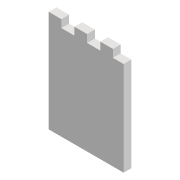
# Autodesk Inventor part: 00_Baseplate_Simmo_side6_v2
Saved by Autodesk Inventor 2022 (Build 260153000, 153)
## iProperties
Created: 2022-08-09
Part Number: 00_Baseplate_Simmo_side6_v2
Material: Generic
Document SubType Name: Modeling
Designer: wanghaoran
Density: 1 g/cm^3
Appearance: Default
Author: wanghaoran
Autodesk Inventor part; units mm, degrees
ref_plane "YZ Plane" through (0, 0, 0) normal (1, 0, 0) x (0, 1, 0)
ref_plane "XZ Plane" through (0, 0, 0) normal (0, 1, 0) x (-1, 0, 0)
ref_plane "XY Plane" through (0, 0, 0) normal (0, 0, 1) x (1, 0, 0)
sketch "Sketch1" plane through (0, 0, 0) normal (0, 0, 1) x (1, 0, 0)
  line L0 (40, 0) -> (48.2654, 0) projected
  line L1 (-10, 0) -> (-10, 6) projected
  line L2 (-10, 0) -> (-10, 6) projected
  line L3 (-10, 0) -> (-10, 6) projected
  line L4 (-10, 6) -> (48.2654, 6)
  line L5 (48.2654, 6) -> (48.2654, -73)
  line L6 (48.2654, -73) -> (-10, -73)
  line L7 (-10, -73) -> (-10, 6)
  point P0 (0, 0)
  dimension "d0" = 79
  constraints: 8 end point, 2 parallel, 1 horizontal, 1 perpendicular
  measures "d0" distance of L4.end L5.end
extrude "Extrusion1" add sketch "Sketch1" along normal blind 6
sketch "Sketch2" plane through (0, 0, 6) normal (0, 0, 1) x (1, 0, 0)
  line L0 (40, 0) -> (48.2654, 0) projected
  line L1 (40, 6) -> (40, 0) projected
  line L2 (48.2654, -73) -> (48.2654, 6) projected
  line L3 (48.2654, 6) -> (-10, 6) projected
  line L4 (20, 6) -> (20, 0) projected
  line L5 (10, 0) -> (10, 6) projected
  line L6 (0, 0) -> (10, 0) projected
  line L7 (0, 6) -> (0, 0) projected
  line L8 (20, 0) -> (30, 0) projected
  line L9 (30, 0) -> (30, 6) projected
  line L10 (40, 0) -> (39.9, 0)
  line L11 (39.9, 0) -> (39.9, 6)
  line L12 (39.9, 6) -> (40, 6)
  line L13 (40, 6) -> (40, 0)
  line L14 (30, 0) -> (30.1, 0)
  line L15 (30.1, 0) -> (30.1, 6)
  line L16 (30.1, 6) -> (30, 6)
  line L17 (30, 6) -> (30, 0)
  line L18 (20, 0) -> (19.9, 0)
  line L19 (19.9, 0) -> (19.9, 6)
  line L20 (19.9, 6) -> (20, 6)
  line L21 (20, 6) -> (20, 0)
  line L22 (10, 0) -> (10.1, 0)
  line L23 (10.1, 0) -> (10.1, 6)
  line L24 (10.1, 6) -> (10, 6)
  line L25 (10, 6) -> (10, 0)
  line L26 (0, 0) -> (-0.1, 0)
  line L27 (-0.1, 0) -> (-0.1, 6)
  line L28 (-0.1, 6) -> (0, 6)
  line L29 (0, 6) -> (0, 0)
  dimension "d3" = 0.1
  dimension "d4" = 6
  dimension "d5" = 0.1
  dimension "d6" = 6
  dimension "d7" = 0.1
  dimension "d8" = 6
  dimension "d9" = 0.1
  dimension "d10" = 6
  dimension "d11" = 0.1
  dimension "d12" = 6
  constraints: 40 end point, 10 parallel, 5 horizontal, 5 perpendicular
  measures "d3" distance of L11.end L12.end
  measures "d4" distance of L10.end L11.end
  measures "d5" distance of L16.end L15.end
  measures "d6" distance of L15.end L14.end
  measures "d7" distance of L19.end L20.end
  measures "d8" distance of L18.end L19.end
  measures "d9" distance of L24.end L23.end
  measures "d10" distance of L23.end L22.end
  measures "d11" distance of L27.end L28.end
  measures "d12" distance of L26.end L27.end
extrude "Extrusion2" cut sketch "Sketch2" against normal blind 6
equation "\"d13\" = d10"
body "Solid1"
